enz one piece 6_v3 (Autodesk Fusion 360 design; units mm, degrees)
Autodesk Fusion 360 part; units mm, degrees
sketch "base" plane through (0, 0, 0) normal (0, 0, 1) x (1, 0, 0)
  circle A0 centre (-22.4, 0.0874) radius 6.2
  circle A1 centre (-22.4, 0.0874) radius 6.8
  circle A2 centre (0, 0) radius 32.25
  circle A3 centre (0, 0) radius 5.6
  circle A4 centre (0, 0) radius 6.2
  circle A5 centre (-15.9191, -15.7337) radius 6.8
  circle A6 centre (-15.9191, -15.7337) radius 6.2
  circle A7 centre (-0.1492, -22.3382) radius 6.8
  circle A8 centre (-0.1492, -22.3382) radius 6.2
  circle A9 centre (15.672, -15.8573) radius 6.8
  circle A10 centre (15.672, -15.8573) radius 6.2
  circle A11 centre (22.2765, -0.0874) radius 6.8
  circle A12 centre (22.2765, -0.0874) radius 6.2
  circle A13 centre (15.7956, 15.7337) radius 6.8
  circle A14 centre (15.7956, 15.7337) radius 6.2
  circle A15 centre (0.0256, 22.3382) radius 6.8
  circle A16 centre (0.0256, 22.3382) radius 6.2
  circle A17 centre (-15.7955, 15.8573) radius 6.8
  circle A18 centre (-15.7955, 15.8573) radius 6.2
  point P0 (-22.4, 0.0874)
  point P1 (-0.0618, 0)
  dimension "d6" = 13.6
  dimension "d54" = 12.4
  dimension "d65" = 360
  dimension "d67" = 22.4
  dimension "d68" = 12.4
  dimension "d69" = 11.2
  constraint concentric A0 A1
  constraint coincident A2.centre A3.centre
  constraint concentric A3 A4
  constraint coincident P0 A0.centre
  measures "d6" diameter of A1
  measures "d54" diameter of A4
  measures "d67" horizontal distance of P0 A2.centre
  measures "d68" diameter of A0
  measures "d69" diameter of A3
extrude "Extrude9" add sketch "base" along normal blind 2 contours A0 | A3 | A6 | A8 | A10 | A12 | A14 | A16 | A18 makes body 1 at (-21.9504, 1.9652, 0) makes body 2 at (-1.1594, 3.2855, 0) makes body 3 at (-1.0077, 24.128, 0) makes body 4 at (-16.0598, -17.6115, 0) makes body 5 at (13.6247, 16.6304, 0) makes body 6 at (-17.3623, 17.9551, 0) makes body 7 at (13.6555, -17.0215, 0) makes body 8 at (23.8739, 1.5284, 0) makes body 9 at (-0.9042, -20.6825, 0)
extrude "seat" add sketch "base" along normal blind 2 from surface at 36 separate body contours A2 makes body 10
extrude "tubes" add sketch "base" along normal blind 38 contours A1 | A4 | A5 | A7 | A9 | A11 | A13 | A15 | A17 bodies 6 4 2 3 9 8 1 5 7 10
sketch "rim" plane through (0, 0, 0) normal (0, 1, 0) x (1, 0, 0)
  line L0 (32.75, -37.2) -> (32.75, -49.2)
  line L1 (32.75, -37.2) -> (29.1786, -37.2)
  line L2 (29.1786, -37.2) -> (29.1786, -49.2)
  line L3 (29.1786, -49.2) -> (32.75, -49.2)
  line L4 (32.75, -49.2) -> (37.1882, -52.2)
  line L5 (29.1786, -49.2) -> (33.6169, -52.2)
  line L6 (33.6169, -52.2) -> (37.1882, -52.2)
  point P0 (32.75, -37.2)
  point P1 (-0.0618, 0)
  dimension "d26" = 37.2
  dimension "d27" = 32.75
  dimension "d29" = 12
  dimension "d35" = 3
  dimension "d37" = 2
  dimension "d61" = 5.357
  dimension "d63" = 37.25
  constraint coincident P0 L0.start
  constraint perpendicular L0 L1
  constraint perpendicular L1 L2
  constraint parallel L1 L3
  constraint equal L4 L5
  constraint parallel L4 L5
  constraint horizontal L6
  measures "d26" vertical distance of origin L0.start
  measures "d27" horizontal distance of P0 origin
  measures "d29" distance of P0 L0.end
  measures "d35" vertical distance of L0.end L4.end
  measures "d37" distance of L4 L5
  measures "d61" distance of L2.end L5.end
  measures "d63" horizontal distance of L4.end P1
revolve "Revolve2" add sketch "rim" angle 360 about axis through (0, 0, 1.75) along (0, 0, 1) bodies 6
sketch "washer mold" plane through (0, 0, 0) normal (0, 0, 1) x (1, 0, 0)
  circle A0 centre (100, 0) radius 19.375
  circle A1 centre (100, 0) radius 16.375
  circle A2 centre (100, 0) radius 15.625
  circle A3 centre (100, 0) radius 18.625
  point P0 (100, 0)
  dimension "d85" = 37.25
  dimension "d86" = 32.75
  dimension "d87" = 38.75
  dimension "d88" = 31.25
  constraint concentric A1 A3
  constraint concentric A2 A3
  constraint concentric A0 A2
  measures "d85" diameter of A3
  measures "d86" diameter of A1
  measures "d87" diameter of A0
  measures "d88" diameter of A2
extrude "Extrude10" add sketch "washer mold" along normal blind 2 separate body contours A3 makes body 11
extrude "Extrude11" add sketch "washer mold" along normal blind 5 bodies 11
equation "d6 = bigTubeOutsideDiameter + tubeWallThickness"
equation "submergedTubeHeight = 36 mm"
equation "capHeightAndOverhead = 12 mm"
equation "bigTubeOutsideDiameter = 12.4 mm"
equation "largeRimOutsideDiameter = 74.5 mm"
equation "baseRimOutsideDiameter = largeRimOutsideDiameter - 9 mm"
equation "generalThickness = 2 mm"
equation "tubeWallThickness = 1.2 mm"
equation "d26 = submergedTubeHeight + tubeWallThickness"
equation "d27 = baseRimOutsideDiameter / 2"
equation "d29 = capHeightAndOverhead"
equation "d37 = generalThickness"
equation "d39 = submergedTubeHeight + tubeBottomThickness"
equation "d42 = submergedTubeHeight + tubeBottomThickness - generalThickness"
equation "d43 = generalThickness"
equation "d51 = tubeBottomThickness"
equation "d54 = smallTubeOutsideDiameter + tubeWallThickness"
equation "smallTubeOutsideDiameter = 11.2 mm"
equation "d63 = largeRimOutsideDiameter / 2"
equation "d65 = 360.0 °"
equation "tubeBottomThickness = 2 mm"
equation "d68 = bigTubeOutsideDiameter"
equation "d69 = smallTubeOutsideDiameter"
equation "j = submergedTubeHeight + tubeBottomThickness - generalThickness"
equation "d85 = largeRimOutsideDiameter / 2"
equation "d86 = ( baseRimOutsideDiameter / 2 mm ) * 1 mm"
equation "d87 = largeRimOutsideDiameter / 2 + 1.5 mm"
equation "d88 = baseRimOutsideDiameter / 2 - 1.5 mm"
named bodies: "holderAndTubes", "washerMold"
